portatermometro (Autodesk Fusion 360 design; units mm, degrees)
Autodesk Fusion 360 part; units mm, degrees
sketch "Sketch1" plane through (0, 0, 0) normal (0, 0, 1) x (1, 0, 0)
  line L0 (22.5, -13) -> (-22.5, -13)
  line L1 (-22.5, -13) -> (-22.5, 13)
  line L2 (-22.5, 13) -> (22.5, 13)
  line L3 (22.5, 13) -> (22.5, -13)
  line L4 (22.5, -13) -> (-22.5, 13) construction
  line L5 (-22.5, -13) -> (22.5, 13) construction
  line L6 (24.9, -15.4) -> (-24.9, -15.4)
  line L7 (-24.9, -15.4) -> (-24.9, 15.4)
  line L8 (-24.9, 15.4) -> (24.9, 15.4)
  line L9 (24.9, 15.4) -> (24.9, -15.4)
  circle A0 centre (-16.6096, 4.1088) radius 4
  dimension "d1" = 45
  dimension "d2" = 26
  dimension "d3" = -2.4
  dimension "d12" = 8
  constraint horizontal L0
  constraint perpendicular L0 L1
  constraint parallel L0 L2
  constraint parallel L1 L3
  constraint coincident L4 origin
  constraint coincident L5 origin
  measures "d1" distance of L1.end L2.end
  measures "d2" distance of L0.end L1.end
  measures "d12" diameter of A0
extrude "Extrude1" add sketch "Sketch1" along normal blind 15 contours L6 L7 L8 L9
sketch "Sketch2" plane through (24.9, 0, 0) normal (1, 0, 0) x (0, 1, 0)
  line L0 (-15.4, 0) -> (15.4, 0)
  line L1 (15.4, 0) -> (15.4, 15)
  line L2 (15.4, 15) -> (-15.4, 15)
  line L3 (-15.4, 15) -> (-15.4, 0)
  line L4 (-15.4, 0) -> (15.4, 0)
  line L5 (15.4, 0) -> (-6.816, -22.216)
  line L6 (-6.816, -22.216) -> (-15.4, 0)
  line L7 (9.6059, -2.4) -> (-5.9061, -17.912)
  line L8 (-5.9061, -17.912) -> (-11.8997, -2.4)
  line L9 (-11.8997, -2.4) -> (9.6059, -2.4)
  dimension "d6" = 45
  dimension "d7" = 2.4
  constraint coincident L0.start L3.end
  constraint coincident L0.end L1.start
  measures "d6" angle of L4 L5
extrude "Extrude2" add sketch "Sketch2" against normal blind 49.8 contours L0 L4 L5 L6
extrude "Extrude3" add sketch "Sketch2" against normal blind 2.4 contours L7 L8 L9
extrude "Extrude4" cut sketch "Sketch1" against normal blind 2.4 contours A0
fillet "Fillet1" radius 5 2 edges at (0, -15.4, 0) (0, 15.4, 0)
fillet "Fillet2" radius 1.2 12 edges at (-24.9, 3.5598, -11.8402) (-24.9, 15.0194, 0.1577) (-24.9, 15.4, 8.5355) (-24.9, -10.94, -11.5428) (-24.9, -15.3153, 0.0158) (-24.9, -15.4, 7.9662) (24.9, -10.94, -11.5428) (24.9, -15.3153, 0.0158) (24.9, -15.4, 7.9662) (24.9, 3.5598, -11.8402) (24.9, 15.0194, 0.1577) (24.9, 15.4, 8.5355)
fillet "Fillet3" radius 1.5 3 edges at (24.5485, -6.6827, -21.5857) (0, -6.816, -22.216) (-24.5485, -6.6827, -21.5857)
